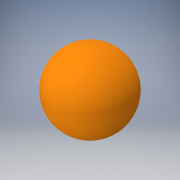
# Autodesk Inventor part: Pelota
Saved by Autodesk Inventor 2016 SP2 (Build 200236200, 236)
## iProperties
Created: 2017-07-03
Part Number: Pelota
Material: Resina fenólica
Document SubType Name: Modeling
Designer: ssant
Density: 1.38 g/cm^3
Appearance: Naranja
Author: ssant
Autodesk Inventor part; units mm, degrees
ref_plane "YZ Plane" through (0, 0, 0) normal (1, 0, 0) x (0, 1, 0)
ref_plane "XZ Plane" through (0, 0, 0) normal (0, 1, 0) x (-1, 0, 0)
ref_plane "XY Plane" through (0, 0, 0) normal (0, 0, 1) x (1, 0, 0)
sketch "Boceto1" plane through (0, 0, 0) normal (0, 0, 1) x (1, 0, 0)
  arc A0 (0, -19.5575) -> (0, 19.5575) centre (0, 0) ccw
  line L0 (0, 0) -> (0, 23.3896)
  line L1 (0, 0) -> (0, -21.567)
  dimension "d0" = 39.115
  constraints: 4 end point, 2 point on circle, 2 point on line, 2 vertical, 1 centre point, 1 coincident
  measures "d0" diameter of A0
revolve "Revolución1" add sketch "Boceto1" angle 360 about axis through (0, 0, 0) along (0, 1, 0)
